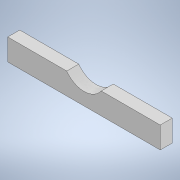
# Autodesk Inventor part: Motor_MainAxis_Fixation
Saved by Autodesk Inventor 2022 (Build 260153000, 153)
## iProperties
Created: 2022-07-26
Part Number: Motor_MainAxis_Fixation
Material: Generisch
Document SubType Name: Modeling
Designer: alexw
Density: 1 g/cm^3
Appearance: Vorgabe
Mass: 29.5996 g
Surface Area: 92.6273 cm^2
Volume: 29.5996 cm^3
Author: alexw
Autodesk Inventor part; units mm, degrees
ref_plane "YZ Plane" through (0, 0, 0) normal (1, 0, 0) x (0, 1, 0)
ref_plane "XZ Plane" through (0, 0, 0) normal (0, 1, 0) x (-1, 0, 0)
ref_plane "XY Plane" through (0, 0, 0) normal (0, 0, 1) x (1, 0, 0)
sketch "Skizze4" plane through (0, 0, 0) normal (0, 0, 1) x (1, 0, 0)
  circle A0 centre (0, 28) radius 17.5 construction
  line L0 (14.3614, 18) -> (63.5, 18)
  line L1 (63.5, 18) -> (63.5, 0)
  line L2 (63.5, 0) -> (-63.5, 0)
  line L3 (-63.5, 0) -> (-63.5, 18)
  line L4 (-63.5, 18) -> (-14.3614, 18)
  arc A1 (-14.3614, 18) -> (14.3614, 18) centre (0, 28) ccw
  line L5 (0, 0) -> (0, 28) construction
  line L6 (-23.5, 56) -> (23.5, 56) construction
  line L7 (23.5, 56) -> (23.5, 0) construction
  line L8 (23.5, 0) -> (-23.5, 0) construction
  line L9 (-23.5, 0) -> (-23.5, 56) construction
  line L10 (-23.5, 56) -> (23.5, 0) construction
  line L11 (23.5, 56) -> (-23.5, 0) construction
  line L12 (-23.5, 41) -> (-8.5, 56) construction
  line L13 (23.5, 41) -> (8.5, 56) construction
  dimension "d37" = 35
  dimension "d38" = 18
  dimension "d39" = 10
  dimension "d40" = 127
  dimension "d43" = 47
  dimension "d44" = 45
  dimension "d45" = 45
  dimension "d46" = 15
  dimension "d47" = 15
  constraints: 28 end point, 6 point on line, 4 perpendicular, 4 point on circle, 3 midpoint, 2 centre point, 2 horizontal, 2 parallel, 1 coincident, 1 collinear, 1 concentric, 1 vertical
  measures "d37" diameter of A0
  measures "d38" distance between parallel lines of L0 L2
  measures "d39" distance from line of A0.centre L0
  measures "d40" distance between parallel lines of L1 L3
  measures "d43" distance between parallel lines of L7 L9
  measures "d44" angle of L6 L13
  measures "d45" angle of L6 L12
  measures "d46" horizontal distance of L12.end L12.start
  measures "d47" horizontal distance of L13.start L13.end
extrude "Extrusion3" add sketch "Skizze4" along normal blind 10
